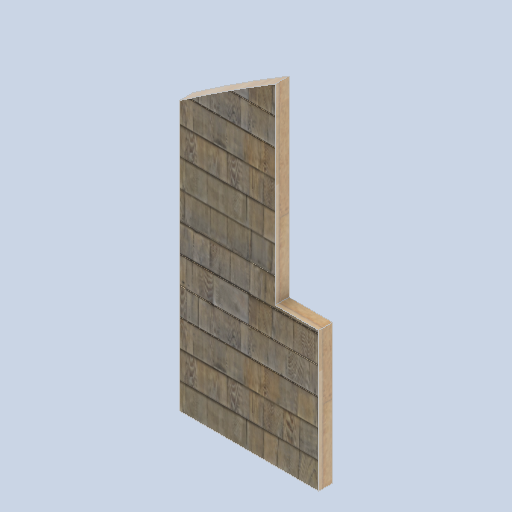
# Autodesk Inventor part: front_wall_block03
Saved by Autodesk Inventor 2024.2 (Build 282272000, 272)
## iProperties
Created: 2024-05-21
Part Number: front_wall_block03
Material: Wood (Maple)
Document SubType Name: Modeling
Designer: LOSTER_1
Density: 0.67 g/cm^3
Appearance: Natural Maple - Glossy Dark Tint
Author: LOSTER_1
Autodesk Inventor part; units mm, degrees
ref_plane "YZ Plane" through (0, 0, 0) normal (1, 0, 0) x (0, 1, 0)
ref_plane "XZ Plane" through (0, 0, 0) normal (0, 1, 0) x (-1, 0, 0)
ref_plane "XY Plane" through (0, 0, 0) normal (0, 0, 1) x (1, 0, 0)
sketch "Sketch1" plane through (0, 0, 0) normal (0, 0, 1) x (1, 0, 0)
  line L0 (-419.0894, 3166.7598) -> (-168.8434, 3166.7598)
  line L1 (-419.0894, 4266.7805) -> (-419.0894, 3166.7598)
  arc A0 (-419.0894, 4266.7805) -> (-968.8434, 3909.8415) centre (4748.6891, -4294.4149) ccw
  line L2 (-968.8434, 2366.6217) -> (-968.8434, 3909.8415)
  line L3 (-168.8434, 2366.6217) -> (-968.8434, 2366.6217)
  line L4 (-168.8434, 3166.7598) -> (-168.8434, 2366.6217)
  constraints: 10 end point, 2 point on circle, 1 centre point, 1 coincident
extrude "Extrusion1" add sketch "Sketch1" along normal blind 80
body "Solid1"
